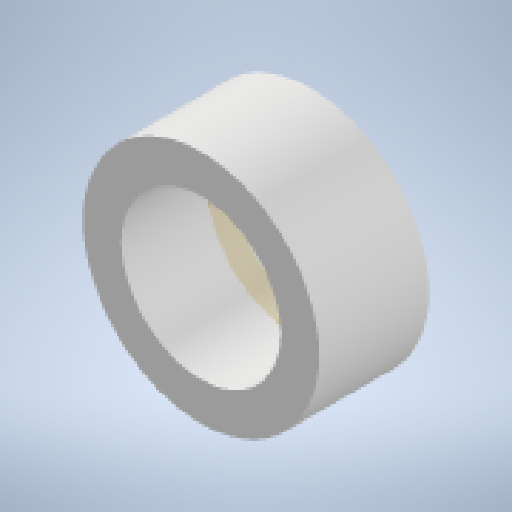
# Autodesk Inventor part: Część4
Saved by Autodesk Inventor 2024 (Build 280153000, 153)
## iProperties
Created: 2023-11-21
Part Number: Część4
Material: Ogólny
Document SubType Name: Modeling
Designer: Wojciech
Density: 1 g/cm^3
Appearance: Domyślna
Author: Wojciech
Autodesk Inventor part; units mm, degrees
ref_plane "YZ Plane" through (0, 0, 0) normal (1, 0, 0) x (0, 1, 0)
ref_plane "XZ Plane" through (0, 0, 0) normal (0, 1, 0) x (-1, 0, 0)
ref_plane "XY Plane" through (0, 0, 0) normal (0, 0, 1) x (1, 0, 0)
ref_plane "Płaszczyzna konstrukcyjna1" through (0, 0, 0) normal (0, 0, 1) x (1, 0, 0)
sketch "Szkic1" plane through (0, 0, 0) normal (0, 0, 1) x (1, 0, 0)
  circle A0 centre (0, 0) radius 52.5 projected
  circle A1 centre (0, 0) radius 35.3896
  constraints: 1 centre point, 1 coincident
extrude "Wyciągnięcie proste1" add sketch "Szkic1" along normal blind 60 and the other way blind 10
